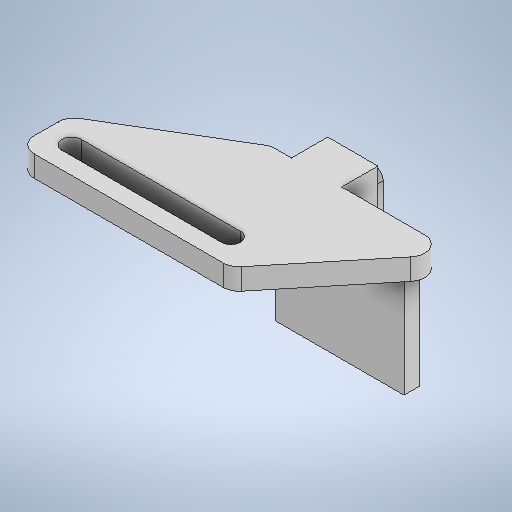
# Autodesk Inventor part: Limit Switch Mount (Left)
Saved by Autodesk Inventor 2025.1 (Build 291241020, 241B)
## iProperties
Created: 2025-01-11
Part Number: Limit Switch Mount (Left)
Material: Generic
Document SubType Name: Modeling
Designer: AtuStem
Density: 1 g/cm^3
Appearance: Default
Author: AtuStem
Autodesk Inventor part; units mm, degrees
ref_plane "YZ Plane" through (0, 0, 0) normal (1, 0, 0) x (0, 1, 0)
ref_plane "XZ Plane" through (0, 0, 0) normal (0, 1, 0) x (-1, 0, 0)
ref_plane "XY Plane" through (0, 0, 0) normal (0, 0, 1) x (1, 0, 0)
sketch "Sketch1" plane through (0, 0, 0) normal (0, 1, 0) x (-1, 0, 0)
  line L0 (0, 0) -> (-42.7482, 0)
  line L1 (-42.7482, 0) -> (-42.7482, -12.7)
  line L2 (-42.7482, -12.7) -> (0, -12.7)
  line L3 (0, -12.7) -> (0, 0)
  line L4 (0, -6.35) -> (-42.7482, -6.35)
  circle A0 centre (-2.286, -6.35) radius 2.286
  circle A1 centre (-40.4622, -6.35) radius 2.286
  line L5 (0, 0) -> (4.064, 0)
  line L6 (4.064, 0) -> (4.064, -12.7)
  line L7 (4.064, -12.7) -> (0, -12.7)
  line L8 (0, -12.7) -> (0, 0)
  line L9 (-42.7482, 0) -> (-46.8122, 0)
  line L10 (-46.8122, 0) -> (-46.8122, -12.7)
  line L11 (-46.8122, -12.7) -> (-42.7482, -12.7)
  line L12 (-42.7482, -12.7) -> (-42.7482, 0)
  line L13 (-2.286, -4.064) -> (-40.4622, -4.064)
  line L14 (-2.286, -8.636) -> (-40.4622, -8.636)
  dimension "d0" = 12.7
  dimension "d1" = 42.7482
  dimension "d2" = 4.572
  dimension "d3" = 4.572
  dimension "d4" = 2.286
  dimension "d5" = 2.286
  dimension "d6" = 4.064
  dimension "d7" = 4.064
  constraints: 30 end point, 7 parallel, 4 point on circle, 3 horizontal, 3 perpendicular, 2 centre point, 2 midpoint, 2 point on line, 1 tangent
  measures "d0" distance of L0.end L1.end
  measures "d1" distance of L1.end L2.end
  measures "d2" diameter of A0
  measures "d3" diameter of A1
  measures "d4" distance from line of L3 A0.centre
  measures "d5" distance from line of L1 A1.centre
  measures "d6" distance between parallel lines of L6 L3
  measures "d7" distance between parallel lines of L10 L1
extrude "Extrusion1" add sketch "Sketch1" along normal blind 5.08 contours L3 A0 L13 A1 L1 L0 | L5 L6 L7 L3 | L1 L11 L10 L9 | L3 L2 L1 A1 L14 A0
sketch "Sketch2" plane through (0, 5.08, 0) normal (0, 1, 0) x (1, 0, 0)
  line L0 (-4.064, 12.7) -> (-4.064, 0) projected
  line L1 (-4.064, 0) -> (46.8122, 0)
  line L2 (46.8122, 0) -> (46.8122, -17.272)
  line L3 (46.8122, -17.272) -> (-4.064, -17.272)
  line L4 (-4.064, -17.272) -> (-4.064, 0)
  point P0 (0, 0)
  point P1 (46.8122, -8.636)
  dimension "d10" = 50.8762
  dimension "d11" = 17.272
  constraints: 8 end point, 2 parallel, 1 horizontal, 1 midpoint, 1 perpendicular
  measures "d10" distance from line of point (46.812, -8.636) L4
  measures "d11" distance between parallel lines of L1 L3
extrude "Extrusion2" add sketch "Sketch2" against normal blind 5.08
sketch "Sketch9" plane through (-4.064, 5.08, 17.272) normal (0, 0, 1) x (1, 0, 0)
  line L0 (66.2305, -31.9278) -> (66.2305, -10.0838)
  line L1 (66.2305, -31.9278) -> (35.4457, -31.9278)
  line L2 (35.4457, -10.0838) -> (35.4457, -31.9278)
  line L3 (44.7294, -25.4988) -> (44.7294, -18.2598)
  arc A0 (40.4492, -25.4988) -> (44.7294, -25.4988) centre (42.5893, -25.4988) ccw
  line L4 (40.4492, -18.2598) -> (40.4492, -25.4988)
  line L5 (44.7294, -13.6878) -> (44.7294, -18.2598)
  line L6 (40.4492, -18.2598) -> (40.4492, -13.6878)
  line L7 (40.4492, -13.6878) -> (40.4492, -6.4488)
  arc A1 (44.7294, -6.4488) -> (40.4492, -6.4488) centre (42.5893, -6.4488) ccw
  line L8 (44.7294, -6.4488) -> (44.7294, -13.6878)
  line L9 (40.4492, -13.6878) -> (44.7294, -13.6878)
  line L10 (44.7294, -18.2598) -> (40.4492, -18.2598)
  arc A2 (71.2343, -5.08) -> (66.2305, -10.0838) centre (71.2343, -10.0838) ccw
  arc A3 (35.4457, -10.0838) -> (30.4419, -5.08) centre (30.4419, -10.0838) ccw
  line L11 (40.8305, -31.9278) -> (66.2305, -31.9278)
  line L12 (29.464, -5.08) -> (71.2343, -5.08)
  line L13 (35.4457, -10.0838) -> (35.4457, -5.08)
  line L14 (66.2305, -10.0838) -> (66.2305, -5.08)
  point P0 (40.9442, -5.08)
  point P1 (30.4419, -5.08)
  point P2 (44.2344, -5.08)
  dimension "d43" = 25.4
  constraints: 30 end point, 8 point on circle, 4 centre point, 3 point on line, 2 horizontal, 1 parallel
  measures "d43" distance of L11.start L11.end
extrude "Extrusion7" add sketch "Sketch9" against normal blind 3.81 contours L1 L2 L13 L12 A1 L7 L6 L4 A0 L3 L5 L8 L14 L0 | L12 A1 | A1 L8 L9 L7 L12 | L3 A0 L4 L10
extrude "Extrusion8" add sketch "Sketch9" along normal blind 12.7 contours L12 A1 | A1 L8 L9 L7 L12 | L3 A0 L4 L10
sketch "Sketch10" plane through (46.8122, 0, 17.272) normal (0, 1, 0) x (1, 0, 0)
  line L0 (15.3543, 5.08) -> (20.3581, 5.08) projected
  line L1 (0, 0) -> (0, 29.972) projected
  line L2 (0, 29.972) -> (20.3581, 5.08)
  line L3 (-15.4305, 0) -> (-20.4343, 0) projected
  line L4 (-20.4343, 0) -> (-50.8762, 18.288)
  line L5 (-50.8762, 29.972) -> (-50.8762, 0) projected
  line L6 (0, 29.972) -> (-0.0381, 3.81)
  line L7 (15.3543, 3.81) -> (-15.4305, 3.81) projected
  line L8 (0, 0) -> (20.3581, 0)
  line L9 (20.3581, 0) -> (20.3581, 5.08)
  line L10 (20.3581, 5.08) -> (0, 5.08)
  line L11 (0, 5.08) -> (0, 0)
  line L12 (-50.8762, 29.972) -> (-50.8762, 0) projected
  line L13 (-50.8762, 18.288) -> (-50.8762, 0)
  line L14 (-50.8762, 0) -> (-20.4343, 0)
  point P0 (-46.8122, 17.272)
  constraints: 18 end point, 2 parallel, 2 perpendicular, 1 horizontal, 1 midpoint, 1 point on line, 1 vertical
extrude "Extrusion9" add sketch "Sketch10" along normal blind 5.08 contours L10 L1 L2 L0 | L0 L9 L8 L1 L10
extrude "Extrusion10" cut sketch "Sketch10" along normal blind 5.08 contours L14 L5 L4
fillet "Fillet4" radius 3.81 6 edges at (46.8122, 2.54, -12.7) (-4.064, 2.54, -12.7) (-4.064, 2.54, -1.016) (26.3779, 2.54, 17.272) (67.1703, 2.54, 12.192) (67.1703, 2.54, 17.272)
fillet "Fillet5" radius 2.54 3 edges at (62.1665, 0, 15.367) (46.7741, 0, 13.462) (31.3817, 0, 15.367)
mirror "Mirror1" about plane through (46.8122, 0, -12.7) normal (0, 0, -1) remove original yes
sketch "Sketch11" plane through (63.287, 5.08, -42.672) normal (0, 0, -1) x (-1, 0, 0)
  line L0 (31.9053, -31.9278) -> (31.9053, -7.62) projected
  line L1 (35.8527, 0) -> (0, 0) projected
  line L2 (31.9053, -31.9278) -> (19.8657, -31.9278)
  line L3 (19.8657, -31.9278) -> (19.8657, 0)
  line L4 (19.8657, 0) -> (31.9053, 0)
  line L5 (31.9053, 0) -> (31.9053, -31.9278)
  point P0 (63.287, -5.08)
  dimension "d54" = 12.0396
  constraints: 8 end point, 2 parallel, 1 horizontal, 1 perpendicular, 1 point on line
  measures "d54" distance between parallel lines of L3 L0
extrude "Extrusion11" add sketch "Sketch11" along normal blind 8.6868
sketch "Sketch12" plane through (63.287, 5.08, -51.3588) normal (0, 0, -1) x (-1, 0, 0)
  line L0 (22.6216, -13.6878) -> (26.9018, -13.6878) projected
  line L1 (26.9018, -13.6878) -> (26.9018, -18.2598) projected
  line L2 (22.6216, -13.6878) -> (26.9018, -13.6878)
  line L3 (26.9018, -13.6878) -> (26.9018, -18.2598)
  line L4 (26.9018, -18.2598) -> (22.6216, -18.2598)
  line L5 (22.6216, -18.2598) -> (22.6216, -13.6878)
  point P0 (63.287, -5.08)
  constraints: 8 end point, 2 parallel, 1 horizontal, 1 perpendicular
extrude "Extrusion12" cut sketch "Sketch12" against normal up to surface (12.4968 mm away)
body "Solid1"
